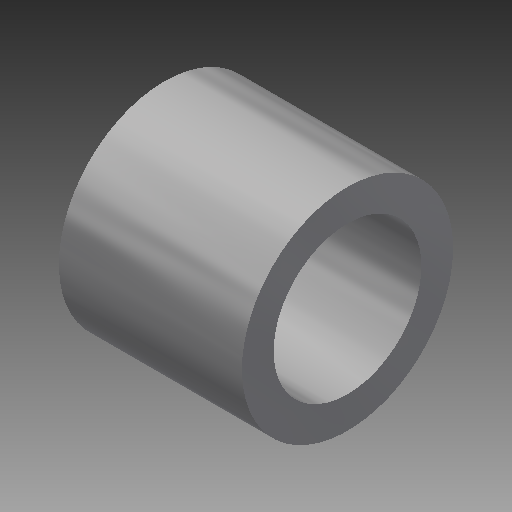
# Autodesk Inventor part: Sleeve
Saved by Autodesk Inventor 2017 (Build 210142000, 142)
## iProperties
Created: 2012-08-06
Part Number: Sleeve
Material: Steel
Document SubType Name: Modeling
Designer: John
Mass: 4.06931 g
Surface Area: 7.09365 cm^2
Volume: 0.518383 cm^3
Density: 7.85 g/cm^3
Appearance: Steel
Author: John
Autodesk Inventor part; units mm, degrees
ref_plane "YZ Plane" through (0, 0, 0) normal (1, 0, 0) x (0, 1, 0)
ref_plane "XZ Plane" through (0, 0, 0) normal (0, 1, 0) x (-1, 0, 0)
ref_plane "XY Plane" through (0, 0, 0) normal (0, 0, 1) x (1, 0, 0)
sketch "Sketch1" plane through (0, 0, 0) normal (1, 0, 0) x (0, 1, 0)
  circle A0 centre (0, 0) radius 5.715
  circle A1 centre (0, 0) radius 4.0005
  dimension "d0" = 11.43
  dimension "d2" = 8.001
  constraints: 2 centre point, 2 coincident
  measures "d0" diameter of A0
  measures "d2" diameter of A1
extrude "Extrusion1" add sketch "Sketch1" along normal blind 9.906
body "Solid1"
